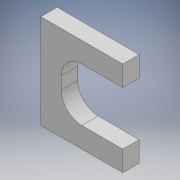
# Autodesk Inventor part: camera strand
Saved by Autodesk Inventor 2017 (Build 210142000, 142)
## iProperties
Created: 2018-12-06
Part Number: camera strand
Material: Generic
Document SubType Name: Modeling
Designer: Eric the Great
Density: 1 g/cm^3
Appearance: Default
Author: Eric the Great
Autodesk Inventor part; units mm, degrees
ref_plane "YZ Plane" through (0, 0, 0) normal (1, 0, 0) x (0, 1, 0)
ref_plane "XZ Plane" through (0, 0, 0) normal (0, 1, 0) x (-1, 0, 0)
ref_plane "XY Plane" through (0, 0, 0) normal (0, 0, 1) x (1, 0, 0)
sketch "Sketch1" plane through (0, 0, 0) normal (0, 1, 0) x (-1, 0, 0)
  line L0 (-7.5, 6.5) -> (2.5, 6.5)
  line L1 (7.5, 1.5) -> (7.5, -1.5)
  line L2 (2.5, -6.5) -> (-7.5, -6.5)
  line L3 (-7.5, -6.5) -> (-7.5, 6.5)
  line L4 (-7.5, 6.5) -> (7.5, -6.5) construction
  line L5 (7.5, 6.5) -> (-7.5, -6.5) construction
  line L6 (12.5, -11.5) -> (12.5, 11.5)
  line L7 (12.5, 11.5) -> (-7.5, 11.5)
  line L8 (-7.5, -11.5) -> (12.5, -11.5)
  line L9 (-7.5, 6.5) -> (-7.5, 11.5)
  line L10 (-7.5, -6.5) -> (-7.5, -11.5)
  arc A0 (7.5, 1.5) -> (2.5, 6.5) centre (2.5, 1.5) ccw
  arc A1 (2.5, -6.5) -> (7.5, -1.5) centre (2.5, -1.5) ccw
  line L11 (0, 0) -> (3.7715, 0)
  dimension "d0" = 15
  dimension "d1" = 13
  dimension "d2" = 5
  dimension "d3" = 5
  dimension "d4" = 5
  constraints: 24 end point, 5 point on line, 4 point on circle, 4 tangent, 3 parallel, 2 centre point, 2 horizontal, 2 midpoint, 2 perpendicular, 1 equal radius, 1 vertical, 1 other
  measures "d0" distance of L4.end L2.end
  measures "d1" distance of L5.start L4.end
  measures "d2" radius of A0
  measures "d3" distance between parallel lines of L7 L0
  measures "d4" distance from line of L1.end L6
extrude "Extrusion1" add sketch "Sketch1" along normal blind 4 contours L9 L7 L6 L8 L10 L2 A1 L1 A0 L0
body "Solid1"
